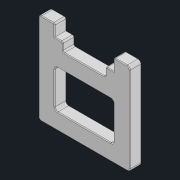
# Autodesk Inventor part: scara-base29
Saved by Autodesk Inventor 2022 (Build 260153000, 153)
## iProperties
Created: 2021-11-05
Part Number: scara-base29
Material: 一般
Document SubType Name: Modeling
Designer: Yuta Kage
Density: 1 g/cm^3
Appearance: 既定
Author: Yuta Kage
Autodesk Inventor part; units mm, degrees
ref_plane "YZ Plane" through (0, 0, 0) normal (1, 0, 0) x (0, 1, 0)
ref_plane "XZ Plane" through (0, 0, 0) normal (0, 1, 0) x (-1, 0, 0)
ref_plane "XY Plane" through (0, 0, 0) normal (0, 0, 1) x (1, 0, 0)
sketch "スケッチ1" plane through (0, 0, 0) normal (0, 0, 1) x (1, 0, 0)
  line L0 (-31, -31) -> (31, -31)
  line L1 (31, -31) -> (31, 31)
  line L2 (31, 31) -> (-31, 31)
  line L3 (-31, 31) -> (-31, -31)
  line L4 (-31, -31) -> (31, 31) construction
  line L5 (31, -31) -> (-31, 31) construction
  point P0 (0, 0)
  dimension "d0" = 62
  dimension "d1" = 62
  constraints: 12 end point, 2 midpoint, 2 parallel, 1 horizontal, 1 perpendicular
  measures "d0" distance of L1.end L2.end
  measures "d1" distance of L2.end L0.start
extrude "押し出し1" add sketch "スケッチ1" along normal mid plane 8
sketch "スケッチ2" plane through (0, 0, 4) normal (0, 0, 1) x (1, 0, 0)
  line L0 (-20, 23) -> (20, 23)
  line L1 (20, 23) -> (20, 31)
  line L2 (20, 31) -> (-20, 31)
  line L3 (-20, 31) -> (-20, 23)
  line L4 (-20, 23) -> (20, 31) construction
  line L5 (20, 23) -> (-20, 31) construction
  line L6 (31, 31) -> (-31, 31) projected
  line L7 (-14.5, 17) -> (14.5, 17)
  line L8 (14.5, 17) -> (14.5, 23)
  line L9 (14.5, 23) -> (-14.5, 23)
  line L10 (-14.5, 23) -> (-14.5, 17)
  line L11 (-14.5, 17) -> (14.5, 23) construction
  line L12 (14.5, 17) -> (-14.5, 23) construction
  point P0 (0, 0)
  point P1 (0, 27)
  point P2 (0, 27)
  point P3 (0, 20)
  point P4 (0, 20)
  point P5 (0, 27)
  point P6 (14.5, 23)
  dimension "d4" = 40
  dimension "d5" = 8
  dimension "d14" = 29
  dimension "d15" = 6
  constraints: 24 end point, 7 midpoint, 4 parallel, 2 horizontal, 2 perpendicular, 2 point on line, 2 vertical alignment
  measures "d4" distance of L1.end L2.end
  measures "d5" distance of L0.end L1.end
  measures "d14" distance of L7.start L7.end
  measures "d15" distance of L9.end L7.start
extrude "押し出し2" cut sketch "スケッチ2" against normal blind 10
sketch "スケッチ3" plane through (0, 0, 4) normal (0, 0, 1) x (1, 0, 0)
  line L0 (-20, -20) -> (20, -20)
  line L1 (20, -20) -> (20, 6)
  line L2 (20, 6) -> (-20, 6)
  line L3 (-20, 6) -> (-20, -20)
  line L4 (-20, -20) -> (20, 6) construction
  line L5 (20, -20) -> (-20, 6) construction
  line L6 (-31, 31) -> (-31, -31) projected
  line L7 (-31, -31) -> (31, -31) projected
  line L8 (14.5, 17) -> (-14.5, 17) projected
  point P0 (0, 0)
  point P1 (0, -7)
  point P2 (0, -7)
  dimension "d10" = 11
  dimension "d11" = 11
  dimension "d16" = 11
  constraints: 12 end point, 3 midpoint, 2 parallel, 1 horizontal, 1 perpendicular, 1 vertical alignment
  measures "d10" distance between parallel lines of L6 L3
  measures "d11" distance between parallel lines of L7 L0
  measures "d16" distance between parallel lines of L8 L2
extrude "押し出し3" cut sketch "スケッチ3" against normal through all
fillet "フィレット2" radius 1 6 edges at (-14.5, 23, 0) (-14.5, 17, 0) (14.5, 17, 0) (14.5, 23, 0) (-20, 31, 0) (20, 31, 0)
fillet "フィレット3" radius 2 4 edges at (-31, 31, 0) (-31, -31, 0) (31, -31, 0) (31, 31, 0)
fillet "フィレット4" radius 2 4 edges at (-20, 6, 0) (-20, -20, 0) (20, -20, 0) (20, 6, 0)
chamfer "面取り1" distance 0.5 angle 45 60 edges at (31, 0, -4) (30.4142, -30.4142, -4) (0, -31, -4) (-30.4142, -30.4142, -4) (-31, 0, -4) (-30.4142, 30.4142, -4) (-25, 31, -4) (-20.2929, 30.7071, -4) (-20, 26.5, -4) (30.4142, 30.4142, -4) (25, 31, -4) (20.2929, 30.7071, -4) (20, 26.5, -4) (31, 0, 4) (30.4142, 30.4142, 4) (25, 31, 4) (20.2929, 30.7071, 4) (20, 26.5, 4) (30.4142, -30.4142, 4) (0, -31, 4) (-30.4142, -30.4142, 4) (-31, 0, 4) (-30.4142, 30.4142, 4) (-25, 31, 4) (-20.2929, 30.7071, 4) (-20, 26.5, 4) (17.75, 23, -4) (14.7929, 22.7071, -4) (14.5, 20, -4) (14.2071, 17.2929, -4) (0, 17, -4) (-14.2071, 17.2929, -4) (-14.5, 20, -4) (-14.7929, 22.7071, -4) (-17.75, 23, -4) (17.75, 23, 4) (14.7929, 22.7071, 4) (14.5, 20, 4) (14.2071, 17.2929, 4) (0, 17, 4) (-14.2071, 17.2929, 4) (-14.5, 20, 4) (-14.7929, 22.7071, 4) (-17.75, 23, 4) (0, 6, 4) (19.4142, 5.4142, 4) (20, -7, 4) (19.4142, -19.4142, 4) (0, -20, 4) (-19.4142, -19.4142, 4) (-20, -7, 4) (-19.4142, 5.4142, 4) (0, -20, -4) (19.4142, -19.4142, -4) (20, -7, -4) (19.4142, 5.4142, -4) (0, 6, -4) (-19.4142, 5.4142, -4) (-20, -7, -4) (-19.4142, -19.4142, -4)
